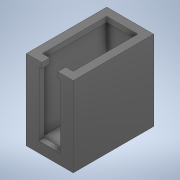
# Autodesk Inventor part: SwitchHolder
Saved by Autodesk Inventor 2020 (Build 240168000, 168)
## iProperties
Created: 2023-12-16
Part Number: SwitchHolder
Material: Thermoplastic Resin
Document SubType Name: Modeling
Designer: smz3rm
Density: 1.28 g/cm^3
Appearance: Smooth - Black
Author: smz3rm
Autodesk Inventor part; units mm, degrees
ref_plane "YZ Plane" through (0, 0, 0) normal (1, 0, 0) x (0, 1, 0)
ref_plane "XZ Plane" through (0, 0, 0) normal (0, 1, 0) x (-1, 0, 0)
ref_plane "XY Plane" through (0, 0, 0) normal (0, 0, 1) x (1, 0, 0)
sketch "Sketch1" plane through (0, 0, 0) normal (0, 1, 0) x (-1, 0, 0)
  line L0 (-3.4, 6.55) -> (3.4, 6.55)
  line L1 (3.4, 6.55) -> (3.4, -6.55)
  line L2 (3.4, -6.55) -> (-3.4, -6.55)
  line L3 (-3.4, -6.55) -> (-3.4, 6.55)
  line L4 (-3.4, 6.55) -> (3.4, -6.55) construction
  line L5 (3.4, 6.55) -> (-3.4, -6.55) construction
  line L6 (4.4, -7.55) -> (4.4, 7.55)
  line L7 (4.4, 7.55) -> (-4.4, 7.55)
  line L8 (-4.4, 7.55) -> (-4.4, -7.55)
  line L9 (-4.4, -7.55) -> (4.4, -7.55)
  point P0 (0, 0)
  dimension "d0" = 6.8
  dimension "d1" = 13.1
  dimension "d2" = 1
  constraints: 20 end point, 4 parallel, 2 midpoint, 2 perpendicular, 1 horizontal, 3 other
  measures "d0" distance of L1.end L2.end
  measures "d1" distance of L0.end L1.end
  measures "d2" distance between parallel lines of L1 L6
extrude "Extrusion1" add sketch "Sketch1" along normal blind 14
sketch "Sketch3" plane through (0, 0, 0) normal (0, -1, 0) x (1, 0, 0)
  line L0 (-4.4, 7.55) -> (4.4, 7.55) projected
  line L1 (-4.4, -7.55) -> (-4.4, 7.55) projected
  line L2 (4.4, -7.55) -> (-4.4, -7.55) projected
  line L3 (4.4, 7.55) -> (4.4, -7.55) projected
  line L4 (-3.4, -6.55) -> (3.4, -6.55) projected
  line L5 (-3.4, 6.55) -> (-3.4, -6.55) projected
  line L6 (3.4, 6.55) -> (-3.4, 6.55) projected
  line L7 (3.4, -6.55) -> (3.4, 6.55) projected
  point P0 (0, 0)
extrude "Extrusion2" add sketch "Sketch3" along normal blind 1 contours L0 L3 L2 L1 | L5 L6 L7 L4
sketch "Sketch4" plane through (-4.4, 14, 7.55) normal (0, 0, 1) x (1, 0, 0)
  line L0 (0, 0) -> (8.8, 0) projected
  line L1 (2.4, 0) -> (6.4, 0)
  line L2 (6.4, 0) -> (6.4, -13)
  line L3 (6.4, -13) -> (2.4, -13)
  line L4 (2.4, -13) -> (2.4, 0)
  point P0 (4.4, -14)
  point P1 (4.4, 0)
  point P2 (4.4, 0)
  point P3 (6.4, 0)
  dimension "d7" = 1
  dimension "d8" = 4
  constraints: 8 end point, 3 midpoint, 2 parallel, 1 horizontal, 1 perpendicular, 1 point on line
  measures "d7" distance from line of point (4.4, -14) L3
  measures "d8" distance between parallel lines of L2 L4
extrude "Extrusion3" cut sketch "Sketch4" against normal up to surface (1 mm away)
sketch "Sketch5" plane through (0, 14, 0) normal (0, 1, 0) x (1, 0, 0)
  line L0 (2, -6.55) -> (2, -7.55) projected
  line L1 (2, -7.55) -> (4.4, -7.55) projected
  line L2 (4.4, -7.55) -> (4.4, 7.55) projected
  line L3 (4.4, 7.55) -> (-4.4, 7.55) projected
  line L4 (-4.4, 7.55) -> (-4.4, -7.55) projected
  line L5 (-4.4, -7.55) -> (-2, -7.55) projected
  line L6 (-2, -7.55) -> (-2, -6.55) projected
  line L7 (-2, -6.55) -> (-3.4, -6.55) projected
  line L8 (-3.4, -6.55) -> (-3.4, 6.55) projected
  line L9 (-3.4, 6.55) -> (3.4, 6.55) projected
  line L10 (3.4, 6.55) -> (3.4, -6.55) projected
  line L11 (3.4, -6.55) -> (2, -6.55) projected
  line L12 (-2.9, 6.05) -> (-2.9, -6.05)
  line L13 (-2.9, -6.05) -> (-1.5, -6.05)
  line L14 (-1.5, -6.05) -> (-1.5, -8.05)
  line L15 (-1.5, -8.05) -> (-4.9, -8.05)
  line L16 (-4.9, -8.05) -> (-4.9, 8.05)
  line L17 (-4.9, 8.05) -> (4.9, 8.05)
  line L18 (4.9, 8.05) -> (4.9, -8.05)
  line L19 (4.9, -8.05) -> (1.5, -8.05)
  line L20 (1.5, -8.05) -> (1.5, -6.05)
  line L21 (1.5, -6.05) -> (2.9, -6.05)
  line L22 (2.9, -6.05) -> (2.9, 6.05)
  line L23 (2.9, 6.05) -> (-2.9, 6.05)
  line L24 (-4.4, -7.55) -> (-2, -7.55) projected
  line L25 (-2, -7.55) -> (-1.5, -7.55)
  line L26 (4.4, -7.55) -> (-4.4, -7.55) projected
  line L27 (2, -7.55) -> (2, -6.55) projected
  line L28 (2, -7.55) -> (1.5, -7.55)
  point P0 (0, 0)
  point P1 (1.5, -7.55)
  dimension "d11" = 0.5
  constraints: 28 end point, 4 point on line, 11 other
  measures "d11" distance between parallel lines of L8 L12
extrude "Extrusion4" add sketch "Sketch5" against normal blind 1 contours L0 L26 L20 L21 L22 L23 L12 L13 L14 L25 L6 L7 L8 L9 L10 L11
body "Solid1"
